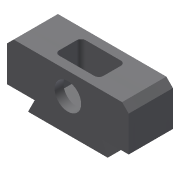
# Autodesk Inventor part: Slider
Saved by Autodesk Inventor 2022 Beta2 (Build 260130000, 130) ContinuousBuild 0
## iProperties
Created: 2011-02-11
Part Number: Slider
Material: Generic
Document SubType Name: Modeling
Designer: landrews
Density: 1 g/cm^3
Appearance: Light Gray
Author: landrews
Autodesk Inventor part; units mm, degrees
ref_plane "YZ Plane" through (0, 0, 0) normal (1, 0, 0) x (0, 1, 0)
ref_plane "XZ Plane" through (0, 0, 0) normal (0, 1, 0) x (-1, 0, 0)
ref_plane "XY Plane" through (0, 0, 0) normal (0, 0, 1) x (1, 0, 0)
sketch "Sketch1" plane through (0, 0, 0) normal (0, 1, 0) x (-1, 0, 0)
  line L0 (-27.5, 6) -> (-15, 6)
  line L1 (-15, 6) -> (-18, 0)
  line L2 (-27.5, 25) -> (-27.5, 6)
  line L3 (-27.5, 25) -> (0, 25)
  line L4 (-18, 0) -> (0, 0)
  line L5 (0, -5) -> (0, 30) projected
  line L6 (38.5, 0) -> (-38.5, 0) projected
  line L7 (27.5, 6) -> (15, 6)
  line L8 (15, 6) -> (18, 0)
  line L9 (27.5, 25) -> (27.5, 6)
  line L10 (27.5, 25) -> (0, 25)
  line L11 (18, 0) -> (0, 0)
  dimension "d9" = 19
  dimension "d10" = 25
  dimension "d11" = 27.5
  dimension "d17" = 12.5
  dimension "d19" = 9.5
  constraints: 20 end point, 4 symmetric about line, 3 point on line, 2 horizontal
  measures "d9" distance of L2.start L0.start
  measures "d10" distance between parallel lines of L4 L3
  measures "d11" distance between parallel lines of L5 L2
  measures "d17" distance of L0.start L0.end
  measures "d19" distance from line of L2 L1.end
extrude "Extrusion1" add sketch "Sketch1" along normal mid plane 20
sketch "Sketch2" plane through (0, -10, 0) normal (0, -1, 0) x (1, 0, 0)
  line L0 (18, 0) -> (-18, 0) projected
  line L1 (-27.5, 25) -> (27.5, 25) projected
  point P0 (0, 0)
  point P1 (0, 15)
  point P2 (0, 0)
  dimension "d20" = 10
  constraints: 1 midpoint, 1 vertical alignment
  measures "d20" distance from line of L1 point (0, 15)
hole "Hole1" at (0, -10, 15) direction (0, 1, 0) diameter 12 depth 10
sketch "Sketch3" plane through (-27.5, 10, 25) normal (0, 0, 1) x (1, 0, 0)
  line L0 (19.5, -16) -> (35.5, -16)
  line L1 (37.5, -14) -> (37.5, -6)
  line L2 (35.5, -4) -> (19.5, -4)
  line L3 (17.5, -6) -> (17.5, -14)
  arc A0 (17.5, -14) -> (19.5, -16) centre (19.5, -14) ccw
  arc A1 (35.5, -16) -> (37.5, -14) centre (35.5, -14) ccw
  arc A2 (37.5, -6) -> (35.5, -4) centre (35.5, -6) ccw
  arc A3 (19.5, -4) -> (17.5, -6) centre (19.5, -6) ccw
  line L4 (-11, -10) -> (66, -10) construction
  line L5 (27.5, 4) -> (27.5, -24) construction
  point P0 (27.5, -10)
  point P1 (27.5, -4)
  point P2 (17.5, -10)
  dimension "d28" = 2
  dimension "d29" = 20
  dimension "d30" = 12
  constraints: 8 end point, 8 point on circle, 8 tangent, 4 centre point, 3 equal radius, 2 midpoint, 2 parallel, 1 horizontal, 1 horizontal alignment, 1 perpendicular, 1 vertical alignment, 2 other
  measures "d28" radius of A0
  measures "d29" distance between parallel lines of L1 L3
  measures "d30" distance between parallel lines of L0 L2
extrude "Extrusion2" cut sketch "Sketch3" against normal blind 16
sketch "Sketch4" plane through (0, 10, 0) normal (0, 1, 0) x (1, 0, 0)
  line L0 (27.5, -25) -> (-27.5, -25) projected
  line L1 (27.5, -6) -> (27.5, -25) projected
  line L2 (-27.5, -25) -> (-27.5, -6) projected
  point P0 (0, 0)
  point P1 (-17.5, -16)
  point P2 (17.5, -16)
  dimension "d37" = 10
  dimension "d38" = 9
  dimension "d39" = 10
  constraints: 1 horizontal alignment
  measures "d37" distance from line of L2 point (-17.5, -16)
  measures "d38" distance from line of L0 point (-17.5, -16)
  measures "d39" distance from line of L1 point (17.5, -16)
hole "Hole2" at (-17.5, 10, 16) at (17.5, 10, 16) direction (0, -1, 0) diameter 4.134 depth 8 tip angle 118 thread size "M5x0.8" class "6H" standard "ANSI Metric M Profile"
chamfer "Chamfer1" distance 3 angle 45 2 edges at (27.5, 0, 25) (-27.5, 0, 25)
equation "\"d39\" = d37"
equation "\"d3\" = 0.5"
equation "\"d4\" = 25"
body "Solid1"
